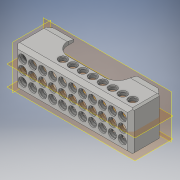
# Autodesk Inventor part: batt_carrier
Saved by Autodesk Inventor 2016 (Build 200138000, 138)
## iProperties
Created: 2016-02-15
Part Number: batt_carrier
Material: Glass
Document SubType Name: Modeling
Designer: jforce
Density: 2.18 g/cm^3
Appearance: Clear
Author: jforce
Autodesk Inventor part; units mm, degrees
ref_plane "YZ Plane" through (0, 0, 0) normal (1, 0, 0) x (0, 1, 0)
ref_plane "XY Plane" through (0, 0, 0) normal (0, 0, 1) x (1, 0, 0)
sketch "Sketch1" plane through (0, 0, 0) normal (0, 0, 1) x (1, 0, 0)
  line L0 (0, 0) -> (70, 0)
  line L1 (70, 0) -> (70, 24)
  line L2 (70, 24) -> (0, 24)
  line L3 (0, 24) -> (0, 0)
  dimension "d0" = 70
  dimension "d1" = 24
  constraints: 8 end point, 2 parallel, 1 horizontal, 1 perpendicular
  measures "d0" distance of L1.end L2.end
  measures "d1" distance of L0.end L1.end
extrude "Extrusion1" add sketch "Sketch1" along normal blind 20.8
chamfer "Chamfer1" distance 1 angle 45 4 edges at (0, 24, 10.4) (70, 24, 10.4) (70, 0, 10.4) (0, 0, 10.4)
chamfer "Chamfer2" distance 2 angle 45 4 edges at (0, 12, 20.8) (35, 0, 20.8) (70, 12, 20.8) (35, 24, 20.8)
shell "Shell1" thickness 2.25 removed faces 1 at (46.3333, 8, 0)
sketch "Sketch2" plane through (1, 0, 0) normal (0, -1, 0) x (1, 0, 0)
  line L0 (51.8009, -2.0517) -> (13.8616, -2.0517)
  line L1 (13.8616, -2.0517) -> (13.8616, 3.4339)
  line L2 (21.8616, 11.4339) -> (43.8009, 11.4339)
  line L3 (51.8009, 3.4339) -> (51.8009, -2.0517)
  arc A0 (51.8009, 3.4339) -> (43.8009, 11.4339) centre (43.8009, 3.4339) ccw
  arc A1 (21.8616, 11.4339) -> (13.8616, 3.4339) centre (21.8616, 3.4339) ccw
  line L4 (70.3236, 4.9809) -> (62.1712, -2.0517)
  line L5 (62.1712, -2.0517) -> (66.7717, -7.3847)
  line L6 (66.7717, -7.3847) -> (74.9241, -0.3522)
  line L7 (74.9241, -0.3522) -> (70.3236, 4.9809)
  line L8 (3.6549, -2.0517) -> (-2.9829, 5.643)
  line L9 (-2.9829, 5.643) -> (-6.2815, 2.7975)
  line L10 (-6.2815, 2.7975) -> (0.3563, -4.8972)
  line L11 (0.3563, -4.8972) -> (3.6549, -2.0517)
  point P0 (-1, 0)
  dimension "d11" = 8
  constraints: 24 end point, 7 parallel, 4 point on circle, 4 tangent, 3 perpendicular, 2 centre point, 1 equal radius, 1 horizontal
  measures "d11" radius of A0
extrude "Extrusion2" cut sketch "Sketch2" against normal through all
chamfer "Chamfer3" distance 4 distance2 1 2 edges at (59.1752, 0, 0) (8.8733, 0, 0) measured on face at (8.8733, 0, 0.5) measured on face at (59.1752, 0, 0.5)
chamfer "Chamfer4" distance 4 distance2 1 2 edges at (8.8733, 24, 0) (59.1752, 24, 0) measured on face at (8.8733, 24, 0.5) measured on face at (59.1752, 24, 0.5)
sketch "Sketch3" plane through (0, 0, 20.8) normal (0, 0, 1) x (1, 0, 0)
  point P0 (0, 0)
  point P1 (64.848, 18.2483)
hole "Hole1" at (64.848, 18.2483, 20.8) direction (0, 0, -1) diameter 4 depth 3 tip angle 118 counterbore diameter 5 counterbore depth 0.85
pattern_linear "Rectangular Pattern1" count 3 spacing 6 along (0, -1, 0) count 11 spacing 6 along (-1, 0, 0) of "Hole1"
sketch "Sketch4" plane through (1, 24, 18.8) normal (0, 1, 0) x (1, 0, 0)
  line L0 (61.848, 0.25) -> (65.848, 0.25) projected
  line L1 (61.848, -1.15) -> (65.848, -1.15) projected
  line L2 (68, 0) -> (0, 0) projected
  line L3 (63.848, 0.25) -> (63.848, 4.25) construction
  point P0 (-1, 18.8)
  dimension "d40" = 4
  constraints: 2 end point, 1 midpoint, 1 vertical
  measures "d40" distance of L3.start L3.end
hole "Hole2" at (64.848, 24, 14.55) direction (0, -1, 0) diameter 4 depth 3 tip angle 118 counterbore diameter 5 counterbore depth 0.85
pattern_linear "Rectangular Pattern2" count 8 spacing 6 along (-1, 0, 0) of "Hole2"
ref_plane "Work Plane3" through (1, 12, 18.8) normal (0, 1, 0) x (1, 0, 0)
mirror "Mirror1" about plane through (1, 12, 18.8) normal (0, 1, 0) of "Hole2", "Rectangular Pattern2"
body "Solid1"
